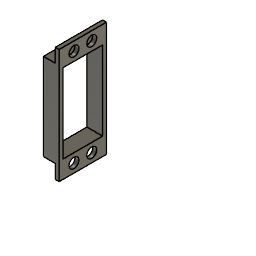
LightServo2 (Autodesk Fusion 360 design; units mm, degrees)
part number: 2026-02-25-22-39-08-175
Autodesk Fusion 360 part; units mm, degrees
sketch "Sketch1" plane through (0, 0, 0) normal (0, 0, 1) x (1, 0, 0)
  line L0 (0, 0) -> (40, 0)
  line L1 (40, 0) -> (40, 20)
  line L2 (40, 20) -> (0, 20)
  line L3 (0, 20) -> (0, 0)
  dimension "d1" = 20
  dimension "d2" = 40
  constraint horizontal L0
  constraint vertical L1
  constraint horizontal L2
  constraint vertical L3
  constraint coincident L0.start L3.end
  measures "d1" distance of L0.start L2.end
  measures "d2" distance of L1.end L2.end
extrude "Extrude1" add sketch "Sketch1" along normal blind 35 makes body 1
sketch "Sketch2" plane through (0, 0, 35) normal (0, 0, 1) x (-1, 0, 0)
  line L0 (0, -20) -> (0, 0)
  line L1 (0, 0) -> (-40, 0)
  line L2 (-40, 0) -> (-40, -20)
  line L3 (-40, -20) -> (0, -20)
  circle A0 centre (-10, -10) radius 3
  line L4 (0, -10) -> (-40, -10) construction
  dimension "d5" = 10
  dimension "d6" = 6
  constraint midpoint L0 L4.start
  constraint midpoint L2 L4.end
  constraint coincident A0.centre L4
  measures "d5" distance of L0 A0.centre
  measures "d6" diameter of A0
extrude "Extrude2" add sketch "Sketch2" along normal blind 4 contours A0 bodies 1
sketch "Sketch3" plane through (0, 0, 0) normal (-1, 0, 0) x (0, -1, 0)
  line L0 (-20, 0) -> (0, 0)
  line L1 (0, 0) -> (0, 35)
  line L2 (0, 35) -> (-20, 35)
  line L3 (-20, 35) -> (-20, 0)
  line L4 (-20, 30) -> (0, 30)
  line L5 (0, 30) -> (0, 28)
  line L6 (0, 28) -> (-20, 28)
  line L7 (-20, 28) -> (-20, 30)
  dimension "d9" = 2
  dimension "d10" = 5
  constraint horizontal L4
  constraint vertical L5
  constraint horizontal L6
  constraint vertical L7
  constraint coincident L1 L5.end
  constraint coincident L3 L4.start
  measures "d9" distance of L4.start L6.end
  measures "d10" distance of L2 L4
extrude "Extrude3" add sketch "Sketch3" along normal blind 7 separate body contours L1 L3 L4 L5 L6 L7 makes body 2
ref_plane "WorkPlane1" through (20, 10, 14) normal (-1, 0, 0) x (0, -1, 0)
mirror "Mirror1" about plane through (20, 10, 14) normal (-1, 0, 0) of bodies 2 makes body 3
combine "Combine1" operation add target body 1 tool bodies 3 2
move_body "Move1" bodies 1 to x (0, 0, -1) y (0, 1, 0) z (1, 0, 0) at (0, 0, 0)
move_body "Move2" bodies 1 to x (-1, 0, 0) y (0, 1, 0) z (0, 0, -1) at (0, 0, 0)
move_body "Move3" bodies 1 to x (1, 0, 0) y (0, 1, 0) z (0, 0, 1) at (0.49, 1.4042, 7.5048)
split "Split1" by plane through (-34.51, 1.4042, 7.5048) normal (-1, 0, 0) bodies 1 makes body 4 at (-35.8434, 11.7029, 14.5197)
ref_plane "WorkPlane2" through (-13.51, 11.4042, 27.5048) normal (0, 0, -1) x (0, -1, 0)
mirror "Mirror2" about plane through (-13.51, 11.4042, 27.5048) normal (0, 0, -1) of bodies 4 makes body 5
delete_body "RemoveBody1" bodies 4
sketch "Sketch4" plane through (-34.51, 0, 0) normal (-1, 0, 0) x (0, -1, 0)
  line L0 (-21.4042, 7.5048) -> (-1.4042, 7.5048)
  line L1 (-1.4042, 7.5048) -> (-1.4042, 47.5048)
  line L2 (-1.4042, 47.5048) -> (-21.4042, 47.5048)
  line L3 (-21.4042, 47.5048) -> (-21.4042, 7.5048)
  line L4 (-23.4042, 56.5048) -> (0.5958, 56.5048)
  line L5 (0.5958, 56.5048) -> (0.5958, -1.4952)
  line L6 (0.5958, -1.4952) -> (-23.4042, -1.4952)
  line L7 (-23.4042, -1.4952) -> (-23.4042, 56.5048)
  line L8 (-1.4042, 54.5048) -> (-21.4042, 54.5048)
  line L9 (-23.4042, 54.5048) -> (0.5958, 54.5048) construction
  line L10 (-1.4042, 0.5048) -> (-21.4042, 0.5048) construction
  dimension "d19" = 2
  dimension "d20" = 2
  dimension "d21" = 2
  dimension "d22" = 2
  constraint horizontal L4
  constraint vertical L5
  constraint horizontal L6
  constraint vertical L7
  constraint coincident L7 L9.start
  constraint coincident L5 L9.end
  constraint perpendicular L5 L9
  constraint coincident L8.end L9
  measures "d19" distance of L3 L7
  measures "d20" distance of L1 L5
  measures "d21" distance of L4 L9
  measures "d22" distance of L6 L10.end
extrude "Extrude4" add sketch "Sketch4" along normal blind 3 and the other way blind 5 separate body makes body 6
sketch "Sketch5" plane through (0.49, 0, 0) normal (1, 0, 0) x (0, 1, 0)
  line L0 (1.4042, 7.5048) -> (21.4042, 7.5048)
  line L1 (21.4042, 7.5048) -> (21.4042, 47.5048)
  line L2 (21.4042, 47.5048) -> (1.4042, 47.5048)
  line L3 (1.4042, 47.5048) -> (1.4042, 7.5048)
  line L4 (-0.5958, -1.4952) -> (23.4042, -1.4952)
  line L5 (23.4042, 56.5048) -> (-0.5958, 56.5048)
  line L6 (-0.5958, 56.5048) -> (-0.5958, -1.4952)
  line L7 (23.4042, -1.4952) -> (23.4042, 56.5048)
  line L8 (-0.5958, 56.5048) -> (23.4042, 56.5048)
  line L9 (23.4042, 56.5048) -> (23.4042, -1.4952)
  line L10 (23.4042, -1.4952) -> (-0.5958, -1.4952)
  line L11 (-0.5958, -1.4952) -> (-0.5958, 56.5048)
  constraint horizontal L8
  constraint vertical L9
  constraint horizontal L10
  constraint vertical L11
  constraint coincident L4.end L7.start
  constraint coincident L5.end L6.start
extrude "Extrude5" add sketch "Sketch5" along normal blind 2 and the other way blind 30 separate body makes body 7
move_body "Move4" bodies 6 to x (1, 0, 0) y (0, 1, 0) z (0, 0, 1) at (-35, 0, 0)
sketch "Sketch6" plane through (2.49, 0, 0) normal (1, 0, 0) x (0, 1, 0)
  line L0 (1.4042, 7.5048) -> (1.4042, 47.5048)
  line L1 (1.4042, 47.5048) -> (21.4042, 47.5048)
  line L2 (21.4042, 47.5048) -> (21.4042, 7.5048)
  line L3 (21.4042, 7.5048) -> (1.4042, 7.5048)
  line L4 (-0.5958, -1.4952) -> (23.4042, -1.4952)
  line L5 (23.4042, -1.4952) -> (23.4042, 56.5048)
  line L6 (23.4042, 56.5048) -> (-0.5958, 56.5048)
  line L7 (-0.5958, 56.5048) -> (-0.5958, -1.4952)
  line L8 (-0.5958, -1.4952) -> (23.4042, -1.4952)
  line L9 (23.4042, -1.4952) -> (23.4042, 5.5048)
  line L10 (23.4042, 5.5048) -> (-0.5958, 5.5048)
  line L11 (-0.5958, 5.5048) -> (-0.5958, -1.4952)
  dimension "d31" = 2
  constraint horizontal L8
  constraint vertical L9
  constraint horizontal L10
  constraint vertical L11
  constraint coincident L5 L9.end
  constraint coincident L4.start L7.end
  measures "d31" distance of L3 L10
extrude "Extrude6" cut sketch "Sketch6" against normal blind 30 contours L4 L5 L7 L8 L9 L10 L11 bodies 7
sketch "Sketch7" plane through (-72.51, 0, 0) normal (-1, 0, 0) x (0, -1, 0)
  line L0 (-21.4042, 7.5048) -> (-21.4042, 47.5048)
  line L1 (-21.4042, 47.5048) -> (-1.4042, 47.5048)
  line L2 (-1.4042, 47.5048) -> (-1.4042, 7.5048)
  line L3 (-1.4042, 7.5048) -> (-21.4042, 7.5048)
  line L4 (-23.4042, -1.4952) -> (0.5958, -1.4952)
  line L5 (0.5958, -1.4952) -> (0.5958, 56.5048)
  line L6 (0.5958, 56.5048) -> (-23.4042, 56.5048)
  line L7 (-23.4042, 56.5048) -> (-23.4042, -1.4952)
  line L8 (-23.4042, -1.4952) -> (0.5958, -1.4952)
  line L9 (0.5958, -1.4952) -> (0.5958, 5.5048)
  line L10 (0.5958, 5.5048) -> (-23.4042, 5.5048)
  line L11 (-23.4042, 5.5048) -> (-23.4042, -1.4952)
  dimension "d34" = 2
  constraint horizontal L8
  constraint vertical L9
  constraint horizontal L10
  constraint vertical L11
  constraint coincident L5 L9.end
  constraint coincident L4.start L7.end
  measures "d34" distance of L3 L10
sketch "Sketch8" plane through (-72.51, 0, 0) normal (-1, 0, 0) x (0, -1, 0)
extrude "Extrude7" cut sketch "Sketch7" against normal blind 6 contours L4 L5 L7 L8 L9 L10 L11 bodies 6
ref_plane "WorkPlane3" through (-28.51, 11.4042, 27.5048) normal (0, 0, -1) x (0, 1, 0)
sketch "Sketch9" plane through (-72.51, 0, 0) normal (-1, 0, 0) x (0, -1, 0)
  line L0 (-23.4042, 5.5048) -> (0.5958, 5.5048)
  line L1 (0.5958, 5.5048) -> (0.5958, 56.5048)
  line L2 (0.5958, 56.5048) -> (-23.4042, 56.5048)
  line L3 (-23.4042, 56.5048) -> (-23.4042, 5.5048)
  line L4 (-21.4042, 7.5048) -> (-21.4042, 47.5048)
  line L5 (-21.4042, 47.5048) -> (-1.4042, 47.5048)
  line L6 (-1.4042, 47.5048) -> (-1.4042, 7.5048)
  line L7 (-1.4042, 7.5048) -> (-21.4042, 7.5048)
  line L8 (-23.4042, 56.5048) -> (0.5958, 56.5048)
  line L9 (0.5958, 56.5048) -> (0.5958, 49.5048)
  line L10 (0.5958, 49.5048) -> (-23.4042, 49.5048)
  line L11 (-23.4042, 49.5048) -> (-23.4042, 56.5048)
  dimension "d37" = 2
  constraint horizontal L8
  constraint vertical L9
  constraint horizontal L10
  constraint vertical L11
  constraint coincident L1 L9.end
  constraint coincident L2.end L3.start
  measures "d37" distance of L5 L10
extrude "Extrude8" cut sketch "Sketch9" against normal blind 6 contours L1 L2 L3 L8 L9 L10 L11 bodies 6
sketch "Sketch10" plane through (2.49, 0, 0) normal (1, 0, 0) x (0, 1, 0)
  line L0 (-0.5958, 5.5048) -> (23.4042, 5.5048)
  line L1 (23.4042, 5.5048) -> (23.4042, 56.5048)
  line L2 (23.4042, 56.5048) -> (-0.5958, 56.5048)
  line L3 (-0.5958, 56.5048) -> (-0.5958, 5.5048)
  line L4 (1.4042, 7.5048) -> (1.4042, 47.5048)
  line L5 (1.4042, 47.5048) -> (21.4042, 47.5048)
  line L6 (21.4042, 47.5048) -> (21.4042, 7.5048)
  line L7 (21.4042, 7.5048) -> (1.4042, 7.5048)
  line L8 (-0.5958, 56.5048) -> (23.4042, 56.5048)
  line L9 (23.4042, 56.5048) -> (23.4042, 49.5048)
  line L10 (23.4042, 49.5048) -> (-0.5958, 49.5048)
  line L11 (-0.5958, 49.5048) -> (-0.5958, 56.5048)
  dimension "d40" = 2
  constraint horizontal L8
  constraint vertical L9
  constraint horizontal L10
  constraint vertical L11
  constraint coincident L1 L9.end
  constraint coincident L2.end L3.start
  measures "d40" distance of L5 L10
extrude "Extrude9" cut sketch "Sketch10" against normal blind 30 contours L1 L2 L3 L8 L9 L10 L11 bodies 7
sketch "Sketch11" plane through (2.49, 0, 0) normal (1, 0, 0) x (0, 1, 0)
  line L0 (1.4042, 7.5048) -> (1.4042, 47.5048)
  line L1 (1.4042, 47.5048) -> (21.4042, 47.5048)
  line L2 (21.4042, 47.5048) -> (21.4042, 7.5048)
  line L3 (21.4042, 7.5048) -> (1.4042, 7.5048)
  line L4 (23.4042, 49.5048) -> (-0.5958, 49.5048)
  line L5 (-0.5958, 49.5048) -> (-0.5958, 5.5048)
  line L6 (-0.5958, 5.5048) -> (23.4042, 5.5048)
  line L7 (23.4042, 5.5048) -> (23.4042, 49.5048)
  line L8 (-0.5958, 49.5048) -> (23.4042, 49.5048)
  line L9 (23.4042, 49.5048) -> (23.4042, 5.5048)
  line L10 (23.4042, 5.5048) -> (-0.5958, 5.5048)
  line L11 (-0.5958, 5.5048) -> (-0.5958, 49.5048)
  constraint horizontal L8
  constraint vertical L9
  constraint horizontal L10
  constraint vertical L11
  constraint coincident L6.end L7.start
  constraint coincident L4.end L5.start
extrude "Extrude10" add sketch "Sketch11" along normal blind 2 contours L0 L1 L2 L3 | L4 L5 L6 L7 L8 L9 L10 L11 bodies 7
sketch "Sketch12" plane through (-27.51, 0, 0) normal (1, 0, 0) x (0, 1, 0)
  line L0 (-0.5958, 49.5048) -> (23.4042, 49.5048)
  line L1 (23.4042, 49.5048) -> (23.4042, 56.5048)
  line L2 (23.4042, 56.5048) -> (-0.5958, 56.5048)
  line L3 (-0.5958, 56.5048) -> (-0.5958, 49.5048)
  circle A0 centre (6.9042, 52.0048) radius 2.5
  line L4 (11.4042, 56.5048) -> (11.4042, 49.5048) construction
  line L5 (2.4042, 56.5048) -> (20.4042, 56.5048) construction
  line L6 (20.4042, 56.5048) -> (20.4042, 49.5048) construction
  line L7 (20.4042, 49.5048) -> (2.4042, 49.5048) construction
  line L8 (2.4042, 49.5048) -> (2.4042, 56.5048) construction
  circle A1 centre (15.9042, 52.0048) radius 2.5
  line L9 (1.4042, 47.5048) -> (21.4042, 47.5048)
  dimension "d45" = 5
  dimension "d49" = 9
  dimension "d50" = 4.5
  dimension "d51" = 4.5
  constraint midpoint L2 L4.start
  constraint midpoint L0 L4.end
  constraint horizontal L5
  constraint vertical L6
  constraint horizontal L7
  constraint vertical L8
  constraint coincident L0 L6.end
  constraint coincident L2 L5.start
  constraint symmetric L4 L6 L8
  constraint symmetric A0 L4 A1
  measures "d45" diameter of A0
  measures "d49" distance of L4 L8
  measures "d50" distance of A0.centre L8
  measures "d51" distance of A1.centre L9
extrude "Extrude11" cut sketch "Sketch12" against normal blind 61 contours A0 | A1 bodies 6 7
split "Split2" by plane through (2.49, 23.4042, 49.5048) normal (0, 0, 1) bodies 7 makes body 8 at (-29.51, 1.0869, 52.8341)
mirror "Mirror3" about plane through (-28.51, 11.4042, 27.5048) normal (0, 0, -1) of bodies 8 makes body 9
sketch "Sketch13" plane through (-27.51, 0, 0) normal (1, 0, 0) x (0, 1, 0)
  line L0 (-0.5958, 5.5048) -> (-0.5958, -1.4952)
  line L1 (-0.5958, -1.4952) -> (23.4042, -1.4952)
  line L2 (23.4042, -1.4952) -> (23.4042, 5.5048)
  line L3 (23.4042, 5.5048) -> (-0.5958, 5.5048)
extrude "Extrude12" cut sketch "Sketch13" against normal blind 15 bodies 7
combine "Combine2" operation add target body 8 tool bodies 7 9
sketch "Sketch14" plane through (-27.51, 0, 0) normal (1, 0, 0) x (0, 1, 0)
  line L0 (23.4042, 5.5048) -> (15.9042, 5.5048)
  circle A0 centre (15.9042, 3.0048) radius 2.5
  line L1 (15.9042, 5.5048) -> (6.9042, 5.5048)
  circle A1 centre (6.9042, 3.0048) radius 2.5
  line L2 (6.9042, 5.5048) -> (-0.5958, 5.5048)
  line L3 (-0.5958, 5.5048) -> (-0.5958, -1.4952)
  line L4 (-0.5958, -1.4952) -> (23.4042, -1.4952)
  line L5 (23.4042, -1.4952) -> (23.4042, 5.5048)
  circle A2 centre (6.9042, 3.0048) radius 2.5
  circle A3 centre (15.9042, 3.0048) radius 2.5
  constraint concentric A1 A2
  constraint concentric A0 A3
extrude "Extrude13" cut sketch "Sketch14" against normal blind 70 contours A0 A3 | A1 A2 bodies 6
combine "Combine3" operation add target body 1 tool bodies 5
hidden bodies 1 8
named bodies: "Servo Model", "Front Servo Cap", "Back Servo Cap"
